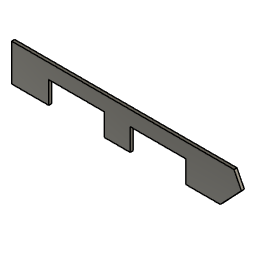
Side Plate v1 (Autodesk Fusion 360 design; units mm, degrees)
Autodesk Fusion 360 part; units mm, degrees
sketch "Sketch1" plane through (0, 0, 0) normal (0, 1, 0) x (1, 0, 0)
  line L0 (0, 0) -> (0, -50)
  line L1 (0, -50) -> (300, -50)
  line L2 (0, 0) -> (50, 0)
  line L3 (50, 0) -> (50, -30)
  line L4 (50, -30) -> (125, -30)
  line L5 (125, -30) -> (125, 0)
  line L6 (125, 0) -> (160, 0)
  line L7 (160, 0) -> (160, -30)
  line L8 (160, -30) -> (235, -30)
  line L9 (235, -30) -> (235, 0)
  line L10 (235, 0) -> (281.5957, 0)
  line L11 (299.4269, -50.5394) -> (300, -50)
  line L12 (0, 0) -> (350, 0) construction
  line L13 (281.5957, 0) -> (310, -30) construction
  line L14 (310, -30) -> (300, -50) construction
  line L15 (281.5957, 0) -> (310, -30)
  line L16 (300, -50) -> (310, -30)
  dimension "d1" = 50
  dimension "d2" = 300
  dimension "d3" = 50
  dimension "d4" = 30
  dimension "d5" = 75
  dimension "d6" = 35
  dimension "d7" = 75
  dimension "d11" = 30
  dimension "d12" = 30
  dimension "d13" = 350
  dimension "d16" = 30
  dimension "d17" = 30
  dimension "d19" = 110
  dimension "d20" = 41.3135
  constraint coincident L0.start L2.start
  constraint vertical L0
  constraint perpendicular L0 L1
  constraint perpendicular L0 L2
  constraint perpendicular L2 L3
  constraint perpendicular L3 L4
  constraint perpendicular L4 L5
  constraint perpendicular L3 L6
  constraint perpendicular L6 L7
  constraint perpendicular L7 L8
  constraint perpendicular L8 L9
  constraint perpendicular L9 L10
  constraint perpendicular L0 L12
  measures "d1" distance of L0.start L0.end
  measures "d2" distance of L0.end L1.end
  measures "d3" distance of L0.start L2.end
  measures "d4" distance of L2.end L3.end
  measures "d5" distance of L3.end L4.end
  measures "d6" distance of L5.end L6.end
  measures "d7" distance of L7.end L8.end
  measures "d11" distance of L8.end L9.end
  measures "d12" distance of L6.end L7.end
  measures "d13" distance of L0.start L12.end
  measures "d16" distance of L4.end L5.end
  measures "d17" vertical distance of L10.end L13.end
  measures "d19" angle of L13 L14
  measures "d20" distance of L10.end L13.end
extrude "Extrude1" add sketch "Sketch1" along normal blind 4
